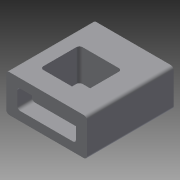
# Autodesk Inventor part: Middle Body
Saved by Autodesk Inventor 2015 (Build 190159000, 159)
## iProperties
Created: 2014-10-29
Part Number: Middle Body
Material: Generic
Document SubType Name: Modeling
Designer: bminden882
Density: 1 g/cm^3
Appearance: Default
Author: bminden882
Autodesk Inventor part; units mm, degrees
ref_plane "YZ Plane" through (0, 0, 0) normal (1, 0, 0) x (0, 1, 0)
ref_plane "XZ Plane" through (0, 0, 0) normal (0, 1, 0) x (-1, 0, 0)
ref_plane "XY Plane" through (0, 0, 0) normal (0, 0, 1) x (1, 0, 0)
sketch "Sketch1" plane through (0, 0, 0) normal (0, 0, 1) x (1, 0, 0)
  line L0 (3.175, 0) -> (80.518, 0)
  line L1 (83.693, 3.175) -> (83.693, 35.433)
  line L2 (80.518, 38.608) -> (3.175, 38.608)
  line L3 (0, 35.433) -> (0, 3.175)
  arc A0 (3.175, 38.608) -> (0, 35.433) centre (3.175, 35.433) ccw
  arc A1 (0, 3.175) -> (3.175, 0) centre (3.175, 3.175) ccw
  arc A2 (80.518, 0) -> (83.693, 3.175) centre (80.518, 3.175) ccw
  arc A3 (83.693, 35.433) -> (80.518, 38.608) centre (80.518, 35.433) ccw
  point P0 (0, 0)
  point P1 (83.693, 38.608)
  point P2 (83.693, 0)
  point P3 (0, 38.608)
  dimension "d0" = 83.693
  dimension "d1" = 38.608
  dimension "d2" = 3.175
  constraints: 8 end point, 8 point on circle, 8 point on line, 8 tangent, 4 centre point, 3 equal radius, 2 parallel, 1 horizontal, 1 perpendicular
  measures "d0" distance of point (0, 38.608) point (83.693, 38.608)
  measures "d1" distance of point (83.693, 38.608) point (83.693, 0)
  measures "d2" radius of A0
extrude "Extrusion1" add sketch "Sketch1" along normal blind 90.043
sketch "Sketch2" plane through (3.175, 38.608, 0) normal (0, 1, 0) x (1, 0, 0)
  line L0 (0, 0) -> (77.343, 0) projected
  line L1 (12.4957, 0) -> (42.2137, 0) construction
  line L2 (0, 0) -> (0, -90.043) projected
  line L3 (77.343, -90.043) -> (0, -90.043) projected
  line L4 (77.343, 0) -> (77.343, -90.043) projected
  line L5 (0, 0) -> (77.343, 0) projected
  line L6 (0, 0) -> (-3.175, 0) projected
  line L7 (80.518, 0) -> (77.343, 0) projected
  line L8 (-3.175, -90.043) -> (0, -90.043) projected
  line L9 (77.343, -90.043) -> (80.518, -90.043) projected
  line L10 (-3.175, 0) -> (-3.175, -90.043) projected
  line L11 (15.621, -29.718) -> (53.34, -29.718)
  line L12 (56.515, -32.893) -> (56.515, -67.31)
  line L13 (53.34, -70.485) -> (15.621, -70.485)
  line L14 (12.446, -67.31) -> (12.446, -32.893)
  arc A0 (15.621, -29.718) -> (12.446, -32.893) centre (15.621, -32.893) ccw
  arc A1 (56.515, -32.893) -> (53.34, -29.718) centre (53.34, -32.893) ccw
  arc A2 (53.34, -70.485) -> (56.515, -67.31) centre (53.34, -67.31) ccw
  arc A3 (12.446, -67.31) -> (15.621, -70.485) centre (15.621, -67.31) ccw
  point P0 (56.515, -70.485)
  point P1 (56.515, -29.718)
  point P2 (12.446, -70.485)
  dimension "d9" = 44.069
  dimension "d10" = 40.767
  dimension "d11" = 15.621
  dimension "d12" = 29.718
  dimension "d13" = 3.175
  constraints: 10 end point, 8 point on circle, 8 tangent, 7 point on line, 4 centre point, 3 equal radius, 2 horizontal, 2 parallel, 1 perpendicular
  measures "d9" distance of point (56.515, -70.485) point (12.446, -70.485)
  measures "d10" distance of point (56.515, -29.718) point (56.515, -70.485)
  measures "d11" distance between parallel lines of L10 L14
  measures "d12" distance between parallel lines of L0 L11
  measures "d13" radius of A0
extrude "Extrusion2" cut sketch "Sketch2" against normal blind 33.02 contours L11 A1 L12 A2 L13 A3 L14 A0
sketch "Sketch3" plane through (0, 0, 90.043) normal (0, 0, 1) x (1, 0, 0)
  line L0 (80.518, 38.608) -> (3.175, 38.608) projected
  line L1 (11.684, 38.608) -> (20.955, 38.608) construction
  line L2 (14.5415, 29.337) -> (69.1515, 29.337)
  line L3 (72.3265, 26.162) -> (72.3265, 12.446)
  line L4 (69.1515, 9.271) -> (14.5415, 9.271)
  line L5 (11.3665, 12.446) -> (11.3665, 26.162)
  arc A0 (14.5415, 29.337) -> (11.3665, 26.162) centre (14.5415, 26.162) ccw
  arc A1 (72.3265, 26.162) -> (69.1515, 29.337) centre (69.1515, 26.162) ccw
  arc A2 (69.1515, 9.271) -> (72.3265, 12.446) centre (69.1515, 12.446) ccw
  arc A3 (11.3665, 12.446) -> (14.5415, 9.271) centre (14.5415, 12.446) ccw
  line L6 (83.693, 3.175) -> (83.693, 35.433) projected
  line L7 (0, 35.433) -> (0, 3.175) projected
  line L8 (3.175, 0) -> (80.518, 0) projected
  point P0 (0, 0)
  point P1 (72.3265, 9.271)
  point P2 (72.3265, 29.337)
  point P3 (11.3665, 9.271)
  dimension "d19" = 60.96
  dimension "d20" = 20.066
  dimension "d21" = 3.175
  dimension "d24" = 11.3665
  dimension "d25" = 9.271
  constraints: 10 end point, 8 point on circle, 8 tangent, 7 point on line, 4 centre point, 3 equal radius, 2 horizontal, 2 parallel, 1 perpendicular
  measures "d19" distance of point (72.326, 9.271) point (11.366, 9.271)
  measures "d20" distance of point (72.326, 29.337) point (72.326, 9.271)
  measures "d21" radius of A0
  measures "d24" distance between parallel lines of L7 L5
  measures "d25" distance between parallel lines of L0 L2
extrude "Extrusion3" cut sketch "Sketch3" against normal blind 15.24
sketch "Sketch4" plane through (0, 0, 0) normal (0, 0, -1) x (-1, 0, 0)
  line L0 (-68.1482, 29.337) -> (-13.5382, 29.337)
  line L1 (-10.3632, 26.162) -> (-10.3632, 12.446)
  line L2 (-13.5382, 9.271) -> (-68.1482, 9.271)
  line L3 (-71.3232, 12.446) -> (-71.3232, 26.162)
  arc A0 (-68.1482, 29.337) -> (-71.3232, 26.162) centre (-68.1482, 26.162) ccw
  arc A1 (-10.3632, 26.162) -> (-13.5382, 29.337) centre (-13.5382, 26.162) ccw
  arc A2 (-13.5382, 9.271) -> (-10.3632, 12.446) centre (-13.5382, 12.446) ccw
  arc A3 (-71.3232, 12.446) -> (-68.1482, 9.271) centre (-68.1482, 12.446) ccw
  line L4 (-3.175, 38.608) -> (-80.518, 38.608) projected
  arc A4 (-80.518, 38.608) -> (-83.693, 35.433) centre (-80.518, 35.433) ccw projected
  line L5 (-83.693, 35.433) -> (-83.693, 3.175) projected
  arc A5 (-83.693, 3.175) -> (-80.518, 0) centre (-80.518, 3.175) ccw projected
  line L6 (-80.518, 0) -> (-3.175, 0) projected
  arc A6 (-3.175, 0) -> (0, 3.175) centre (-3.175, 3.175) ccw projected
  line L7 (0, 3.175) -> (0, 35.433) projected
  arc A7 (0, 35.433) -> (-3.175, 38.608) centre (-3.175, 35.433) ccw projected
  point P0 (0, 0)
  point P1 (-10.3632, 9.271)
  point P2 (-10.3632, 29.337)
  point P3 (-71.3232, 9.271)
  dimension "d28" = 60.96
  dimension "d29" = 20.066
  dimension "d30" = 3.175
  dimension "d31" = 10.3632
  dimension "d32" = 9.271
  constraints: 8 end point, 8 point on circle, 8 tangent, 6 point on line, 4 centre point, 3 equal radius, 2 parallel, 1 horizontal, 1 perpendicular
  measures "d28" distance of point (-10.363, 9.271) point (-71.323, 9.271)
  measures "d29" distance of point (-10.363, 29.337) point (-10.363, 9.271)
  measures "d30" radius of A0
  measures "d31" distance between parallel lines of L7 L1
  measures "d32" distance between parallel lines of L4 L0
extrude "Extrusion5" cut sketch "Sketch4" against normal blind 15.24 contours L0 A1 L1 A2 L2 A3 L3 A0
body "Solid1"
